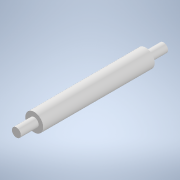
# Autodesk Inventor part: 传动轴2
Saved by Autodesk Inventor 2022 (Build 260153000, 153)
## iProperties
Created: 2023-02-24
Part Number: 传动轴2
Material: 常规
Document SubType Name: Modeling
Designer: 李承轩
Density: 1 g/cm^3
Appearance: 默认
Author: 李承轩
Autodesk Inventor part; units mm, degrees
ref_plane "YZ Plane" through (0, 0, 0) normal (1, 0, 0) x (0, 1, 0)
ref_plane "XZ Plane" through (0, 0, 0) normal (0, 1, 0) x (-1, 0, 0)
ref_plane "XY Plane" through (0, 0, 0) normal (0, 0, 1) x (1, 0, 0)
sketch "草图1" plane through (0, 0, 0) normal (0, 0, 1) x (1, 0, 0)
  circle A0 centre (0, 0) radius 10
  dimension "d0" = 20
  constraints: 1 centre point, 1 coincident
  measures "d0" diameter of A0
extrude "拉伸1" add sketch "草图1" along normal blind 40
sketch "草图2" plane through (0, 0, 40) normal (0, 0, 1) x (1, 0, 0)
  circle A0 centre (0, 0) radius 20 projected
  point P0 (0, 0)
extrude "拉伸2" add sketch "草图2" along normal blind 250
sketch "草图3" plane through (0, 0, 290) normal (0, 0, 1) x (1, 0, 0)
  circle A0 centre (0, 0) radius 10
  dimension "d5" = 20
  constraints: 1 centre point, 1 coincident
  measures "d5" diameter of A0
extrude "拉伸3" add sketch "草图3" along normal blind 40
